Autodesk Inventor part; units mm, degrees
(part 2 of 2)
sketch "Sketch28" plane through (2.5, 0, 0) normal (1, 0, 0) x (0, 0, -1)
  line L0 (82, 17.8) -> (82, 5) projected
  line L1 (66, 17.8) -> (82, 17.8) projected
  line L2 (66, 5) -> (66, 17.8) projected
  line L3 (82, 5) -> (66, 5) projected
  line L4 (67.0532, 35.5) -> (67.0532, 21.8) projected
  line L5 (71.0532, 21.8) -> (71.0532, 35.5) projected
  line L6 (67.0532, 21.8) -> (63.0532, 21.8) projected
  line L7 (63.0532, 21.8) -> (63.0532, 35.5) projected
  line L8 (63.0532, 35.5) -> (67.0532, 35.5) projected
  line L9 (71.0532, 35.5) -> (75.0532, 35.5) projected
  line L10 (75.0532, 35.5) -> (75.0532, 21.8) projected
  line L11 (75.0532, 21.8) -> (71.0532, 21.8) projected
  line L12 (83.0532, 21.8) -> (79.0532, 21.8) projected
  line L13 (79.0532, 21.8) -> (79.0532, 35.5) projected
  line L14 (83.0532, 35.5) -> (83.0532, 21.8) projected
  line L15 (79.0532, 35.5) -> (83.0532, 35.5) projected
  line L16 (59.0532, 5.5) -> (55.0532, 5.5) projected
  line L17 (59.0532, 35.5) -> (59.0532, 5.5) projected
  line L18 (55.0532, 5.5) -> (55.0532, 35.5) projected
  line L19 (55.0532, 35.5) -> (59.0532, 35.5) projected
  line L20 (47.0532, 5.5) -> (47.0532, 35.5) projected
  line L21 (51.0532, 35.5) -> (51.0532, 5.5) projected
  line L22 (51.0532, 5.5) -> (47.0532, 5.5) projected
  line L23 (47.0532, 35.5) -> (51.0532, 35.5) projected
  line L24 (39.0532, 35.5) -> (43.0532, 35.5) projected
  line L25 (43.0532, 5.5) -> (39.0532, 5.5) projected
  line L26 (39.0532, 5.5) -> (39.0532, 35.5) projected
  line L27 (43.0532, 35.5) -> (43.0532, 5.5) projected
  point P0 (0, 0)
extrude "Extrusion27" add sketch "Sketch28" against normal up to surface (5 mm away) contours L0 L3 L2 L1 | L4 L6 L7 L8 | L5 L9 L10 L11 | L12 L13 L15 L14 | L16 L18 L19 L17 | L20 L23 L21 L22
sketch "Sketch29" plane through (2.5, 0, 0) normal (1, 0, 0) x (0, 0, -1)
  line L0 (15.0532, 35.5) -> (19.0532, 35.5) projected
  line L1 (19.0532, 35.5) -> (19.0532, 5.5) projected
  line L2 (19.0532, 5.5) -> (15.0532, 5.5) projected
  line L3 (15.0532, 5.5) -> (15.0532, 35.5) projected
  line L4 (31.0532, 35.5) -> (35.0532, 35.5) projected
  line L5 (35.0532, 35.5) -> (35.0532, 5.5) projected
  line L6 (35.0532, 5.5) -> (31.0532, 5.5) projected
  line L7 (31.0532, 5.5) -> (31.0532, 35.5) projected
  line L8 (23.0532, 35.5) -> (27.0532, 35.5) projected
  line L9 (27.0532, 35.5) -> (27.0532, 5.5) projected
  line L10 (27.0532, 5.5) -> (23.0532, 5.5) projected
  line L11 (23.0532, 5.5) -> (23.0532, 35.5) projected
  line L12 (39.0532, 35.5) -> (43.0532, 35.5) projected
  line L13 (43.0532, 35.5) -> (43.0532, 5.5) projected
  line L14 (43.0532, 5.5) -> (39.0532, 5.5) projected
  line L15 (39.0532, 5.5) -> (39.0532, 35.5) projected
  line L16 (87.0532, 35.5) -> (91.0532, 35.5) projected
  line L17 (91.0532, 35.5) -> (91.0532, 5.5) projected
  line L18 (91.0532, 5.5) -> (87.0532, 5.5) projected
  line L19 (87.0532, 5.5) -> (87.0532, 35.5) projected
  line L20 (95.0532, 35.5) -> (99.0532, 35.5) projected
  line L21 (99.0532, 35.5) -> (99.0532, 5.5) projected
  line L22 (99.0532, 5.5) -> (95.0532, 5.5) projected
  line L23 (95.0532, 5.5) -> (95.0532, 35.5) projected
  circle A0 centre (-30, 10) radius 2.6 projected
  circle A1 centre (-10, 10) radius 2.6 projected
  circle A2 centre (-10, 30) radius 2.6 projected
  circle A3 centre (-30, 30) radius 2.6 projected
  line L24 (112.7, 40) -> (-40, 40) projected
  line L25 (-40, 40) -> (-40, 0) projected
  line L26 (-40, 0) -> (124.7, 0) projected
  line L27 (124.7, 0) -> (124.7, 30.6) projected
  line L28 (124.7, 30.6) -> (112.7, 30.6) projected
  line L29 (112.7, 30.6) -> (112.7, 40) projected
  line L30 (43.0532, 20) -> (58.0532, 20)
  line L31 (58.0532, 20) -> (58.0532, 5)
  line L32 (58.0532, 5) -> (43.0532, 5)
  line L33 (43.0532, 5) -> (43.0532, 20)
  point P0 (0, 0)
  dimension "d199" = 0
  dimension "d200" = 15
  dimension "d201" = 15
  dimension "d202" = 5
  constraints: 8 end point, 2 parallel, 1 horizontal, 1 perpendicular
  measures "d199" distance between parallel lines of L13 L33
  measures "d200" distance of L30.start L30.end
  measures "d201" distance of L30.end L31.end
  measures "d202" distance between parallel lines of L26 L32
extrude "Extrusion28" cut sketch "Sketch29" against normal blind 10 contours L30 L31 L32 L33 L13
sketch "Sketch30" plane through (2.5, 0, 0) normal (1, 0, 0) x (0, 0, -1)
  line L0 (112.7, 40) -> (-40, 40) projected
  line L1 (-40, 40) -> (-40, 0) projected
  line L2 (-40, 0) -> (124.7, 0) projected
  line L3 (124.7, 0) -> (124.7, 30.6) projected
  line L4 (124.7, 30.6) -> (112.7, 30.6) projected
  line L5 (112.7, 30.6) -> (112.7, 40) projected
  circle A0 centre (-30, 30) radius 2.6 projected
  circle A1 centre (-10, 30) radius 2.6 projected
  circle A2 centre (-10, 10) radius 2.6 projected
  circle A3 centre (-30, 10) radius 2.6 projected
  line L6 (95.0532, 35.5) -> (99.0532, 35.5) projected
  line L7 (99.0532, 35.5) -> (99.0532, 5.5) projected
  line L8 (99.0532, 5.5) -> (95.0532, 5.5) projected
  line L9 (95.0532, 5.5) -> (95.0532, 35.5) projected
  line L10 (87.0532, 35.5) -> (91.0532, 35.5) projected
  line L11 (91.0532, 35.5) -> (91.0532, 5.5) projected
  line L12 (91.0532, 5.5) -> (87.0532, 5.5) projected
  line L13 (87.0532, 5.5) -> (87.0532, 35.5) projected
  line L14 (43.0532, 20) -> (58.0532, 20) projected
  line L15 (58.0532, 20) -> (58.0532, 5) projected
  line L16 (58.0532, 5) -> (43.0532, 5) projected
  line L17 (43.0532, 5) -> (43.0532, 5.5) projected
  line L18 (43.0532, 5.5) -> (39.0532, 5.5) projected
  line L19 (39.0532, 5.5) -> (39.0532, 35.5) projected
  line L20 (39.0532, 35.5) -> (43.0532, 35.5) projected
  line L21 (43.0532, 35.5) -> (43.0532, 20) projected
  line L22 (23.0532, 35.5) -> (27.0532, 35.5) projected
  line L23 (27.0532, 35.5) -> (27.0532, 5.5) projected
  line L24 (27.0532, 5.5) -> (23.0532, 5.5) projected
  line L25 (23.0532, 5.5) -> (23.0532, 35.5) projected
  line L26 (31.0532, 35.5) -> (35.0532, 35.5) projected
  line L27 (35.0532, 35.5) -> (35.0532, 5.5) projected
  line L28 (35.0532, 5.5) -> (31.0532, 5.5) projected
  line L29 (31.0532, 5.5) -> (31.0532, 35.5) projected
  line L30 (15.0532, 35.5) -> (19.0532, 35.5) projected
  line L31 (19.0532, 35.5) -> (19.0532, 5.5) projected
  line L32 (19.0532, 5.5) -> (15.0532, 5.5) projected
  line L33 (15.0532, 5.5) -> (15.0532, 35.5) projected
  line L34 (39.0532, 35.5) -> (43.0532, 35.5)
  line L35 (43.0532, 35.5) -> (43.0532, 5.5)
  line L36 (43.0532, 5.5) -> (39.0532, 5.5)
  line L37 (39.0532, 5.5) -> (39.0532, 35.5)
  point P0 (0, 0)
  constraints: 8 end point, 2 parallel, 1 horizontal, 1 perpendicular
extrude "Extrusion29" add sketch "Sketch30" against normal up to surface (5 mm away) contours L35 L18 L19 L20 L21
sketch "Sketch31" plane through (2.5, 0, 0) normal (1, 0, 0) x (0, 0, -1)
  line L0 (112.7, 40) -> (-40, 40) projected
  line L1 (-40, 40) -> (-40, 0) projected
  line L2 (-40, 0) -> (124.7, 0) projected
  line L3 (124.7, 0) -> (124.7, 30.6) projected
  line L4 (124.7, 30.6) -> (112.7, 30.6) projected
  line L5 (112.7, 30.6) -> (112.7, 40) projected
  circle A0 centre (-30, 30) radius 2.6 projected
  circle A1 centre (-10, 30) radius 2.6 projected
  circle A2 centre (-10, 10) radius 2.6 projected
  circle A3 centre (-30, 10) radius 2.6 projected
  line L6 (95.0532, 35.5) -> (99.0532, 35.5) projected
  line L7 (99.0532, 35.5) -> (99.0532, 5.5) projected
  line L8 (99.0532, 5.5) -> (95.0532, 5.5) projected
  line L9 (95.0532, 5.5) -> (95.0532, 35.5) projected
  line L10 (87.0532, 35.5) -> (91.0532, 35.5) projected
  line L11 (91.0532, 35.5) -> (91.0532, 5.5) projected
  line L12 (91.0532, 5.5) -> (87.0532, 5.5) projected
  line L13 (87.0532, 5.5) -> (87.0532, 35.5) projected
  line L14 (43.0532, 20) -> (58.0532, 20) projected
  line L15 (58.0532, 20) -> (58.0532, 5) projected
  line L16 (58.0532, 5) -> (43.0532, 5) projected
  line L17 (43.0532, 5) -> (43.0532, 20) projected
  line L18 (23.0532, 35.5) -> (27.0532, 35.5) projected
  line L19 (27.0532, 35.5) -> (27.0532, 5.5) projected
  line L20 (27.0532, 5.5) -> (23.0532, 5.5) projected
  line L21 (23.0532, 5.5) -> (23.0532, 35.5) projected
  line L22 (31.0532, 35.5) -> (35.0532, 35.5) projected
  line L23 (35.0532, 35.5) -> (35.0532, 5.5) projected
  line L24 (35.0532, 5.5) -> (31.0532, 5.5) projected
  line L25 (31.0532, 5.5) -> (31.0532, 35.5) projected
  line L26 (15.0532, 35.5) -> (19.0532, 35.5) projected
  line L27 (19.0532, 35.5) -> (19.0532, 5.5) projected
  line L28 (19.0532, 5.5) -> (15.0532, 5.5) projected
  line L29 (15.0532, 5.5) -> (15.0532, 35.5) projected
  line L30 (83.0532, 35.5) -> (79.0532, 35.5) projected
  line L31 (83.0532, 5.5) -> (79.0532, 5.5)
  line L32 (79.0532, 5.5) -> (79.0532, 35.5)
  line L33 (79.0532, 35.5) -> (83.0532, 35.5)
  line L34 (83.0532, 35.5) -> (83.0532, 5.5)
  line L35 (75.0532, 35.5) -> (71.0532, 35.5)
  line L36 (71.0532, 35.5) -> (71.0532, 5.5)
  line L37 (71.0532, 5.5) -> (75.0532, 5.5)
  line L38 (75.0532, 5.5) -> (75.0532, 35.5)
  line L39 (67.0532, 35.5) -> (63.0532, 35.5)
  line L40 (63.0532, 35.5) -> (63.0532, 5.5)
  line L41 (63.0532, 5.5) -> (67.0532, 5.5)
  line L42 (67.0532, 5.5) -> (67.0532, 35.5)
  line L43 (59.0532, 35.5) -> (55.0532, 35.5)
  line L44 (55.0532, 35.5) -> (55.0532, 24)
  line L45 (55.0532, 24) -> (59.0532, 24)
  line L46 (59.0532, 24) -> (59.0532, 35.5)
  line L47 (51.0532, 24) -> (47.0532, 24)
  line L48 (47.0532, 24) -> (47.0532, 35.5)
  line L49 (47.0532, 35.5) -> (51.0532, 35.5)
  line L50 (51.0532, 35.5) -> (51.0532, 24)
  line L51 (43.0532, 24) -> (39.0532, 24)
  line L52 (39.0532, 24) -> (39.0532, 35.5)
  line L53 (39.0532, 35.5) -> (43.0532, 35.5)
  line L54 (43.0532, 35.5) -> (43.0532, 24)
  point P0 (0, 0)
  dimension "d207" = 4
  dimension "d208" = 4
  dimension "d209" = 4
  dimension "d210" = 4
  dimension "d211" = 4
  dimension "d212" = 4
  dimension "d213" = 4
  dimension "d214" = 4
  dimension "d215" = 0
  dimension "d216" = 4
  dimension "d217" = 4
  dimension "d218" = 4
  dimension "d219" = 4
  dimension "d220" = 4
  constraints: 48 end point, 12 parallel, 7 point on line, 6 horizontal, 6 perpendicular
  measures "d207" distance of L32.end L33.end
  measures "d208" distance of L37.end L36.end
  measures "d209" distance of L41.end L40.end
  measures "d210" distance between parallel lines of L13 L34
  measures "d211" distance between parallel lines of L38 L32
  measures "d212" distance between parallel lines of L36 L42
  measures "d213" distance of L45.end L44.end
  measures "d214" distance between parallel lines of L14 L45
  measures "d215" distance between parallel lines of L39 L43
  measures "d216" distance of L48.end L49.end
  measures "d217" distance of L52.end L53.end
  measures "d218" distance between parallel lines of L50 L44
  measures "d219" distance between parallel lines of L54 L48
  measures "d220" distance between parallel lines of L40 L46
extrude "Extrusion30" cut sketch "Sketch31" against normal blind 10 contours L34 L31 L32 L30 | L38 L37 L36 L35 | L42 L41 L40 L39 | L46 L45 L44 L43 | L47 L48 L49 L50 | L51 L52 L53 L54
sketch "Sketch33" plane through (0, 2, 0) normal (0, 1, 0) x (1, 0, 0)
  line L0 (-11, 124.7) -> (-11, 107.2) projected
  line L1 (-11, 124.7) -> (-113, 124.7) projected
  line L2 (-113, 107.2) -> (-113, 124.7) projected
  arc A0 (-116, 104.2) -> (-113, 107.2) centre (-116, 107.2) ccw projected
  line L3 (-121.5, 104.2) -> (-116, 104.2) projected
  line L4 (-121.5, 11.25) -> (-121.5, 104.2) projected
  line L5 (-116, 11.25) -> (-121.5, 11.25) projected
  arc A1 (-113, 8.25) -> (-116, 11.25) centre (-116, 8.25) ccw projected
  line L6 (-113, 2.5) -> (-113, 8.25) projected
  line L7 (-11, 2.5) -> (-113, 2.5) projected
  line L8 (-11, 8.25) -> (-11, 2.5) projected
  arc A2 (-8, 11.25) -> (-11, 8.25) centre (-8, 8.25) ccw projected
  line L9 (-2.5, 11.25) -> (-8, 11.25) projected
  line L10 (-2.5, 104.2) -> (-2.5, 11.25) projected
  line L11 (-8, 104.2) -> (-2.5, 104.2) projected
  arc A3 (-11, 107.2) -> (-8, 104.2) centre (-8, 107.2) ccw projected
  circle A4 centre (-27.9, 26.9) radius 1.35
  circle A5 centre (-27.9, 26.9) radius 3.5
  circle A6 centre (-103.9, 26.9) radius 3.5
  circle A7 centre (-103.9, 26.9) radius 1.35
  line L12 (-2.5, 112.7) -> (-2.5, 2.5) projected
  line L13 (-2.5, 2.5) -> (-121.5, 2.5) projected
  line L14 (-121.5, 112.7) -> (-121.5, 2.5) projected
  line L15 (-121.5, 112.7) -> (-124, 112.7) projected
  line L16 (-124, 0) -> (-124, 112.7) projected
  line L17 (0, 0) -> (-124, 0) projected
  line L18 (0, 0) -> (0, -40) projected
  line L19 (0, -40) -> (2.5, -40) projected
  line L20 (2.5, 112.7) -> (2.5, -40) projected
  line L21 (2.5, 112.7) -> (-2.5, 112.7) projected
  point P0 (0, 0)
  dimension "d234" = 2.7
  dimension "d235" = 7
  dimension "d236" = 7
  dimension "d237" = 2.7
  dimension "d238" = 30.4
  dimension "d239" = 76
  dimension "d240" = 97.8
  dimension "d241" = 97.8
  constraints: 4 centre point, 2 coincident
  measures "d234" diameter of A4
  measures "d235" diameter of A5
  measures "d236" diameter of A6
  measures "d237" diameter of A7
  measures "d238" distance from line of L20 A4.centre
  measures "d239" distance of A7.centre A4.centre
  measures "d240" distance from line of L1 A6.centre
  measures "d241" distance from line of L1 A5.centre
extrude "Extrusion32" add sketch "Sketch33" along normal blind 3 contours A5 | A6
sketch "Sketch34" plane through (0, 2, 0) normal (0, 1, 0) x (1, 0, 0)
  circle A0 centre (-27.9, 26.9) radius 3.5 projected
  circle A1 centre (-103.9, 26.9) radius 3.5 projected
  line L0 (-11, 124.7) -> (-11, 107.2) projected
  line L1 (-11, 124.7) -> (-113, 124.7) projected
  line L2 (-113, 107.2) -> (-113, 124.7) projected
  arc A2 (-116, 104.2) -> (-113, 107.2) centre (-116, 107.2) ccw projected
  line L3 (-121.5, 104.2) -> (-116, 104.2) projected
  line L4 (-121.5, 11.25) -> (-121.5, 104.2) projected
  line L5 (-116, 11.25) -> (-121.5, 11.25) projected
  arc A3 (-113, 8.25) -> (-116, 11.25) centre (-116, 8.25) ccw projected
  line L6 (-113, 2.5) -> (-113, 8.25) projected
  line L7 (-11, 2.5) -> (-113, 2.5) projected
  line L8 (-11, 8.25) -> (-11, 2.5) projected
  arc A4 (-8, 11.25) -> (-11, 8.25) centre (-8, 8.25) ccw projected
  line L9 (-2.5, 11.25) -> (-8, 11.25) projected
  line L10 (-2.5, 104.2) -> (-2.5, 11.25) projected
  line L11 (-8, 104.2) -> (-2.5, 104.2) projected
  arc A5 (-11, 107.2) -> (-8, 104.2) centre (-8, 107.2) ccw projected
  circle A6 centre (-103.9, 26.9) radius 1.35 projected
  circle A7 centre (-27.9, 26.9) radius 1.35 projected
  point P0 (0, 0)
extrude "Extrusion33" cut sketch "Sketch34" against normal blind 1 contours A6 | A7
sketch "Sketch35" plane through (2.5, 0, 0) normal (1, 0, 0) x (0, 0, -1)
  line L0 (71.0532, 5.5) -> (71.0532, 35.5) projected
  line L1 (71.0532, 35.5) -> (75.0532, 35.5) projected
  line L2 (75.0532, 35.5) -> (75.0532, 5.5) projected
  line L3 (75.0532, 5.5) -> (71.0532, 5.5) projected
  line L4 (43.0532, 35.5) -> (43.0532, 24) projected
  line L5 (43.0532, 24) -> (39.0532, 24) projected
  line L6 (39.0532, 24) -> (39.0532, 35.5) projected
  line L7 (39.0532, 35.5) -> (43.0532, 35.5) projected
  line L8 (55.0532, 24) -> (55.0532, 35.5) projected
  line L9 (55.0532, 35.5) -> (59.0532, 35.5) projected
  line L10 (59.0532, 35.5) -> (59.0532, 24) projected
  line L11 (59.0532, 24) -> (55.0532, 24) projected
  line L12 (51.0532, 35.5) -> (51.0532, 24) projected
  line L13 (51.0532, 24) -> (47.0532, 24) projected
  line L14 (47.0532, 24) -> (47.0532, 35.5) projected
  line L15 (47.0532, 35.5) -> (51.0532, 35.5) projected
  line L16 (83.0532, 35.5) -> (83.0532, 5.5) projected
  line L17 (83.0532, 5.5) -> (79.0532, 5.5) projected
  line L18 (79.0532, 5.5) -> (79.0532, 35.5) projected
  line L19 (79.0532, 35.5) -> (83.0532, 35.5) projected
  line L20 (63.0532, 5.5) -> (63.0532, 35.5) projected
  line L21 (63.0532, 35.5) -> (67.0532, 35.5) projected
  line L22 (67.0532, 35.5) -> (67.0532, 5.5) projected
  line L23 (67.0532, 5.5) -> (63.0532, 5.5) projected
  line L24 (112.7, 40) -> (-40, 40) projected
  line L25 (-40, 40) -> (-40, 0) projected
  line L26 (-40, 0) -> (124.7, 0) projected
  line L27 (124.7, 0) -> (124.7, 30.6) projected
  line L28 (124.7, 30.6) -> (112.7, 30.6) projected
  line L29 (112.7, 30.6) -> (112.7, 40) projected
  circle A0 centre (-30, 30) radius 2.6 projected
  circle A1 centre (-10, 30) radius 2.6 projected
  circle A2 centre (-10, 10) radius 2.6 projected
  circle A3 centre (-30, 10) radius 2.6 projected
  line L30 (95.0532, 35.5) -> (99.0532, 35.5) projected
  line L31 (99.0532, 35.5) -> (99.0532, 5.5) projected
  line L32 (99.0532, 5.5) -> (95.0532, 5.5) projected
  line L33 (95.0532, 5.5) -> (95.0532, 35.5) projected
  line L34 (87.0532, 35.5) -> (91.0532, 35.5) projected
  line L35 (91.0532, 35.5) -> (91.0532, 5.5) projected
  line L36 (91.0532, 5.5) -> (87.0532, 5.5) projected
  line L37 (87.0532, 5.5) -> (87.0532, 35.5) projected
  line L38 (43.0532, 20) -> (58.0532, 20) projected
  line L39 (58.0532, 20) -> (58.0532, 5) projected
  line L40 (58.0532, 5) -> (43.0532, 5) projected
  line L41 (43.0532, 5) -> (43.0532, 20) projected
  line L42 (23.0532, 35.5) -> (27.0532, 35.5) projected
  line L43 (27.0532, 35.5) -> (27.0532, 5.5) projected
  line L44 (27.0532, 5.5) -> (23.0532, 5.5) projected
  line L45 (23.0532, 5.5) -> (23.0532, 35.5) projected
  line L46 (31.0532, 35.5) -> (35.0532, 35.5) projected
  line L47 (35.0532, 35.5) -> (35.0532, 5.5) projected
  line L48 (35.0532, 5.5) -> (31.0532, 5.5) projected
  line L49 (31.0532, 5.5) -> (31.0532, 35.5) projected
  line L50 (15.0532, 35.5) -> (19.0532, 35.5) projected
  line L51 (19.0532, 35.5) -> (19.0532, 5.5) projected
  line L52 (19.0532, 5.5) -> (15.0532, 5.5) projected
  line L53 (15.0532, 5.5) -> (15.0532, 35.5) projected
  line L54 (112.7, 40) -> (-40, 40)
  line L55 (-40, 40) -> (-40, 0)
  line L56 (-40, 0) -> (112.7, 0)
  line L57 (112.7, 0) -> (112.7, 40)
  point P0 (0, 0)
  constraints: 8 end point, 2 parallel, 1 horizontal, 1 perpendicular
extrude "Extrusion34" cut sketch "Sketch35" against normal blind 5 contours L29 L57 L26 L25 L24
sketch "Sketch36" plane through (-2.5, 0, 0) normal (1, 0, 0) x (0, 0, -1)
  line L0 (0, 0) -> (0, 40) projected
  line L1 (112.7, 0) -> (0, 0) projected
  line L2 (112.7, 30.6) -> (112.7, 0) projected
  line L3 (112.7, 37.5) -> (112.7, 30.6) projected
  line L4 (112.7, 37.5) -> (104.2, 37.5) projected
  line L5 (104.2, 2) -> (104.2, 37.5) projected
  line L6 (104.2, 2) -> (11.25, 2) projected
  line L7 (11.25, 37.5) -> (11.25, 2) projected
  line L8 (11.25, 37.5) -> (2.5, 37.5) projected
  line L9 (2.5, 40) -> (2.5, 37.5) projected
  line L10 (0, 40) -> (2.5, 40) projected
  circle A0 centre (108.45, 27.5) radius 1.35
  circle A1 centre (108.45, 10) radius 1.35
  circle A2 centre (6.875, 27.5) radius 1.35
  circle A3 centre (6.875, 10) radius 1.35
  dimension "d249" = 2.7
  dimension "d250" = 2.7
  dimension "d251" = 2.7
  dimension "d252" = 2.7
  dimension "d253" = 10
  dimension "d254" = 10
  dimension "d255" = 10
  dimension "d256" = 0
  dimension "d259" = 4.25
  constraints: 4 centre point
  measures "d249" diameter of A0
  measures "d250" diameter of A1
  measures "d251" diameter of A2
  measures "d252" diameter of A3
  measures "d253" distance from line of L8 A2.centre
  measures "d254" distance from line of L1 A3.centre
  measures "d255" distance from line of L1 A1.centre
  measures "d256" vertical distance of A2.centre A0.centre
  measures "d259" distance from line of L3 A0.centre
extrude "Extrusion35" cut sketch "Sketch36" against normal blind 6 contours A0 | A1 | A2 | A3
sketch "Sketch37" plane through (-124, 0, -124.7) normal (-1, 0, 0) x (0, 0, 1)
  line L0 (12, 30.6) -> (0, 30.6) projected
  line L1 (0, 0) -> (0, 30.6) projected
  line L2 (0, 0) -> (124.7, 0) projected
  line L3 (124.7, 0) -> (124.7, 40) projected
  line L4 (124.7, 40) -> (12, 40) projected
  line L5 (12, 40) -> (12, 30.6) projected
  line L6 (29.6468, 35.5) -> (29.6468, 5.5) projected
  line L7 (29.6468, 5.5) -> (25.6468, 5.5) projected
  line L8 (25.6468, 5.5) -> (25.6468, 35.5) projected
  line L9 (25.6468, 35.5) -> (29.6468, 35.5) projected
  line L10 (37.6468, 35.5) -> (37.6468, 5.5) projected
  line L11 (37.6468, 5.5) -> (33.6468, 5.5) projected
  line L12 (33.6468, 5.5) -> (33.6468, 35.5) projected
  line L13 (33.6468, 35.5) -> (37.6468, 35.5) projected
  line L14 (53.6468, 35.5) -> (53.6468, 5.5) projected
  line L15 (53.6468, 5.5) -> (49.6468, 5.5) projected
  line L16 (49.6468, 5.5) -> (49.6468, 35.5) projected
  line L17 (49.6468, 35.5) -> (53.6468, 35.5) projected
  line L18 (45.6468, 35.5) -> (45.6468, 5.5) projected
  line L19 (45.6468, 5.5) -> (41.6468, 5.5) projected
  line L20 (41.6468, 5.5) -> (41.6468, 35.5) projected
  line L21 (41.6468, 35.5) -> (45.6468, 35.5) projected
  line L22 (113.45, 4) -> (60, 4) projected
  line L23 (60, 4) -> (60, 32.5785) projected
  line L24 (60, 32.5785) -> (113.45, 32.5785) projected
  line L25 (113.45, 32.5785) -> (113.45, 4) projected
  line L26 (25.6468, 35.5) -> (53.6468, 35.5)
  line L27 (53.6468, 35.5) -> (53.6468, 5.5)
  line L28 (53.6468, 5.5) -> (25.6468, 5.5)
  line L29 (25.6468, 5.5) -> (25.6468, 35.5)
  point P0 (124.7, 0)
  constraints: 8 end point, 2 parallel, 1 horizontal, 1 perpendicular
extrude "Extrusion36" add sketch "Sketch37" against normal blind 2.5 contours L26 L12 L28 L6 | L6 L7 L8 L9 | L13 L10 L11 L12 | L26 L20 L28 L10 | L21 L18 L19 L20 | L26 L16 L28 L18 | L17 L14 L15 L16
sketch "Sketch38" plane through (0, 2, 0) normal (0, 1, 0) x (1, 0, 0)
  line L0 (-11, 124.7) -> (-11, 107.2) projected
  line L1 (-11, 124.7) -> (-113, 124.7) projected
  line L2 (-113, 107.2) -> (-113, 124.7) projected
  arc A0 (-116, 104.2) -> (-113, 107.2) centre (-116, 107.2) ccw projected
  line L3 (-121.5, 104.2) -> (-116, 104.2) projected
  line L4 (-121.5, 11.25) -> (-121.5, 104.2) projected
  line L5 (-116, 11.25) -> (-121.5, 11.25) projected
  arc A1 (-113, 8.25) -> (-116, 11.25) centre (-116, 8.25) ccw projected
  line L6 (-113, 2.5) -> (-113, 8.25) projected
  line L7 (-11, 2.5) -> (-113, 2.5) projected
  line L8 (-11, 8.25) -> (-11, 2.5) projected
  arc A2 (-8, 11.25) -> (-11, 8.25) centre (-8, 8.25) ccw projected
  line L9 (-2.5, 11.25) -> (-8, 11.25) projected
  line L10 (-2.5, 104.2) -> (-2.5, 11.25) projected
  line L11 (-8, 104.2) -> (-2.5, 104.2) projected
  arc A3 (-11, 107.2) -> (-8, 104.2) centre (-8, 107.2) ccw projected
  circle A4 centre (-103.9, 26.9) radius 1.35
  circle A5 centre (-36.9, 26.9) radius 1.35
  circle A6 centre (-103.9, 26.9) radius 3.5
  circle A7 centre (-36.9, 26.9) radius 3.5
  circle A8 centre (-103.9, 26.9) radius 3.5 projected
  circle A9 centre (-27.9, 26.9) radius 3.5 projected
  point P0 (0, 0)
  dimension "d266" = 2.7
  dimension "d267" = 67
  dimension "d269" = 2.7
  dimension "d271" = 7
  dimension "d272" = 7
  dimension "d278" = 0
  dimension "d279" = 0
  dimension "d280" = 0
  constraints: 4 centre point, 2 coincident
  measures "d266" diameter of A5
  measures "d267" distance of A4.centre A5.centre
  measures "d269" diameter of A4
  measures "d271" diameter of A6
  measures "d272" diameter of A7
  measures "d278" distance of A8.centre A6.centre
  measures "d279" vertical distance of A9.centre A7.centre
  measures "d280" distance of A8.centre A6.centre
extrude "Extrusion37" add sketch "Sketch38" along normal blind 3 contours A6 | A7
sketch "Sketch39" plane through (-103.9, 5, -26.9) normal (0, 1, 0) x (1, 0, 0)
  circle A0 centre (67, 0) radius 1.35 projected
  circle A1 centre (67, 0) radius 3.5 projected
  circle A2 centre (0, 0) radius 1.35 projected
  circle A3 centre (0, 0) radius 3.5 projected
  point P0 (103.9, -26.9)
extrude "Extrusion38" cut sketch "Sketch39" against normal blind 4 contours A0 | A2
body "Solid1"
